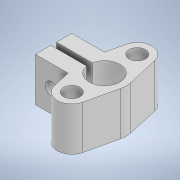
# Autodesk Inventor part: Kep_Truc
Saved by Autodesk Inventor 2022 (Build 260153000, 153)
## iProperties
Created: 2022-11-14
Part Number: Kep_Truc
Material: Generic
Document SubType Name: Modeling
Designer: nguye
Density: 1 g/cm^3
Appearance: Default
Author: nguye
Autodesk Inventor part; units mm, degrees
ref_plane "YZ Plane" through (0, 0, 0) normal (1, 0, 0) x (0, 1, 0)
ref_plane "XZ Plane" through (0, 0, 0) normal (0, 1, 0) x (-1, 0, 0)
ref_plane "XY Plane" through (0, 0, 0) normal (0, 0, 1) x (1, 0, 0)
sketch "Sketch1" plane through (0, 0, 0) normal (0, 1, 0) x (-1, 0, 0)
  circle A0 centre (0, 0) radius 4.25
  circle A1 centre (0, 0) radius 6
  line L0 (14, 5) -> (14, -5)
  line L1 (4.1833, 0.75) -> (14, 0.75)
  line L2 (14, 0.75) -> (14, -0.75)
  line L3 (14, -0.75) -> (4.1833, -0.75)
  circle A2 centre (0, 9) radius 2.25
  circle A3 centre (0, -9) radius 2.25
  circle A4 centre (0, 9) radius 4
  circle A5 centre (0, -9) radius 4
  line L4 (3.9, 9.8889) -> (5.85, 1.3333)
  line L5 (-3.9, 9.8889) -> (-5.85, 1.3333)
  line L6 (5.85, -1.3333) -> (3.9, -9.8889)
  line L7 (-5.85, -1.3333) -> (-3.9, -9.8889)
  line L8 (3.3166, -5) -> (14, -5)
  line L9 (14, 5) -> (3.3166, 5)
  line L10 (18, 0) -> (-10, 0) projected
  point P0 (14, 0)
  point P1 (14, -0.75)
  point P2 (14, 0.75)
  point P3 (5.0143, -5)
  point P4 (5.0143, 5)
  point P5 (5.9529, -0.75)
  point P6 (6, 0)
  point P7 (14, 0)
  dimension "d0" = 8.5
  dimension "d1" = 12
  dimension "d2" = 10
  dimension "d3" = 14
  dimension "d4" = 1.5
  dimension "d5" = 14
  dimension "d6" = 4.5
  dimension "d7" = 4.5
  dimension "d8" = 18
  dimension "d9" = 9
  dimension "d10" = 8
  dimension "d11" = 8
  dimension "d30" = 5
  constraints: 20 end point, 12 point on circle, 7 tangent, 6 centre point, 4 coincident, 4 perpendicular, 2 parallel, 2 vertical alignment, 1 horizontal, 1 horizontal alignment, 1 midpoint
  measures "d0" diameter of A0
  measures "d1" diameter of A1
  measures "d2" distance of L0.start L0.end
  measures "d3" distance from line of point (0, 0) L0
  measures "d4" distance between parallel lines of L3 L1
  measures "d5" distance of point (14, 0) point (0, 0)
  measures "d6" diameter of A2
  measures "d7" diameter of A3
  measures "d8" distance of A3.centre A2.centre
  measures "d9" distance of point (0, 0) A3.centre
  measures "d10" diameter of A4
  measures "d11" diameter of A5
  measures "d30" distance between parallel lines of L10 L8
extrude "Extrusion1" add sketch "Sketch1" along normal blind 12 contours A0 L10 A1 A4 L1 | L3 A1 A5 L10 A0 | A1 L4 L9 L0 L1 | L3 L0 L8 L6 A1 | A1 L9 L4 | L6 L8 A1 | L5 A4 A1 | A1 A5 L7 | A1 A4 L4 L9 | L8 L6 A5 A1 | A4 A1 | A1 A4 | A5 A1 | A1 A5
sketch "Sketch4" plane through (-14, 0, 5) normal (0, 0, 1) x (1, 0, 0)
  line L0 (0, 0) -> (8.9857, 0) projected
  line L1 (0, 12) -> (8.9857, 12) projected
  point P0 (14, 0)
  point P1 (4.5, 6)
  dimension "d31" = 6
  dimension "d32" = 6
  dimension "d33" = 4.5
  measures "d31" distance from line of L0 point (4.5, 6)
  measures "d32" distance from line of L1 point (4.5, 6)
  measures "d33" horizontal distance of L0.start point (4.5, 6)
hole "Hole1" at (-9.5, 6, 5) direction (0, 0, -1) diameter 3.5 depth 10
equation "\"d12\" = d1"
body "Solid1"
